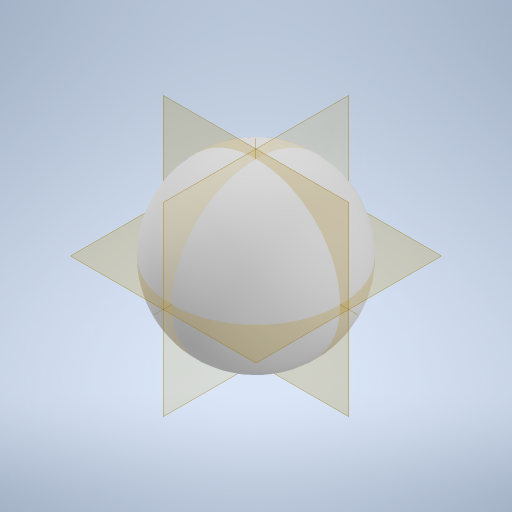
# Autodesk Inventor part: InventorSphere
Saved by Autodesk Inventor 2024 (Build 280153000, 153)
## iProperties
Created: 2024-05-29
Part Number: InventorSphere
Material: Generic
Document SubType Name: Modeling
Designer: jbwk
Density: 1 g/cm^3
Appearance: Default
Author: jbwk
Autodesk Inventor part; units mm, degrees
sketch "Sketch2" plane through (0, 0, 0) normal (0, 0, 1) x (1, 0, 0)
  arc A0 (0, 0.5) -> (0, -0.5) centre (0, 0) ccw
  line L0 (0, 0) -> (0, 1.0772)
  line L1 (0, 1.0772) -> (0, -1.006)
  dimension "d1" = 1
  constraints: 4 end point, 3 point on line, 2 point on circle, 1 centre point, 1 coincident, 1 vertical
  measures "d1" diameter of A0
revolve "Revolution1" add sketch "Sketch2" angle 360 about axis through (0, 1.0772, 0) along (0, -1, 0)
body "Solid1"
